Autodesk Inventor part; units mm, degrees
(part 2 of 3)
sketch "Sketch16" plane through (0, 0, -20.23) normal (0, 0, -1) x (-1, 0, 0)
  line L0 (-4.8, 72.125) -> (14.7092, 72.125) construction
  line L1 (-4.8, 51.125) -> (24.7153, 51.125) construction
  line L2 (17.4444, 66.6309) -> (14.7092, 72.125) construction
  line L3 (14.2591, 61.0912) -> (17.4444, 66.6309) construction
  line L4 (20.0758, 56.9365) -> (14.2591, 61.0912) construction
  line L5 (16.752, 54.0974) -> (20.0758, 56.9365) construction
  line L6 (24.7153, 51.125) -> (16.752, 54.0974) construction
  circle A0 centre (-4.8, 5) radius 1.375 construction
  line L7 (-126.5, -2.5) -> (2.5, -2.5) construction
  line L8 (0.5, -0.5) -> (-124.5, -0.5) construction
  line L9 (0.5, -0.5) -> (-124.5, -0.5) construction
  line L10 (-124, 0) -> (0, 0) construction
  line L11 (-124, 0) -> (0, 0) construction
  line L12 (-124, 0) -> (0, 0) construction
  line L13 (0, 0) -> (-122, 0) construction
  line L14 (-122, -0.5) -> (0.5, -0.5) construction
  line L15 (-98.5, 5) -> (-4.8, 5) construction
  line L16 (2.5, 17.7927) -> (-87.0105, 17.7927) construction
  line L17 (2.5, 14.2427) -> (2.5, 16.7927) construction
  line L18 (2.5, 16.7927) -> (2.5, 11.6927) construction
  line L19 (2.5, 10.6927) -> (-87.0105, 10.6927) construction
  line L20 (-37, 78) -> (-37, 22) construction
  line L21 (-40.5, 25.5) -> (-37, 25.5) construction
  line L22 (-40.5, 25.5) -> (-40.5, 74.5) construction
  circle A1 centre (-40.5, 74.5) radius 1.375 construction
  line L23 (-98.5, 25.5) -> (-98.5, 74.5) construction
  line L24 (-42.1, 82.811) -> (-42.1, 78) construction
  line L25 (-122, 78) -> (0, 78) construction
  line L26 (0, 78) -> (-124, 78) construction
  line L27 (2.5, 83.5) -> (-126.5, 83.5) construction
  line L28 (-124.5, 81.5) -> (0.5, 81.5) construction
  line L29 (-124.5, 81.5) -> (0.5, 81.5) construction
  line L30 (0, 81) -> (-124, 81) construction
  line L31 (0, 81) -> (-124, 81) construction
  line L32 (0, 81) -> (-124, 81) construction
  line L33 (-124, 81) -> (0, 81) construction
  line L34 (-124, 81.5) -> (0, 81.5) construction
  line L35 (0, 81) -> (-124, 81) construction
  line L36 (-40.5, 22) -> (-40.5, 25.5) construction
  circle A2 centre (-40.5, 25.5) radius 1.375 construction
  line L37 (-37, 25.5) -> (-37, 22) construction
  line L38 (-37, 22) -> (-40.5, 22) construction
  line L39 (-37, 22) -> (-122, 22) construction
  line L40 (-40.5, 25.5) -> (-98.5, 25.5) construction
  circle A3 centre (-98.5, 74.5) radius 1.375 construction
  line L41 (-122, 78) -> (-124, 78) construction
  line L42 (-122, 22) -> (-122, 78) construction
  line L43 (-98.5, 74.5) -> (-98.5, 5) construction
  line L44 (-124, 81) -> (-124, 0) construction
  line L45 (-124, 81) -> (-124, 0) construction
  line L46 (-122, 0) -> (-122, 78) construction
  line L47 (-124, 78) -> (-124, 0) construction
  line L48 (-124, 78) -> (-124, 81) construction
  line L49 (-124, 81.5) -> (-124.5, 81.5) construction
  line L50 (2.5, 16.7927) -> (2.5, 17.7927) construction
  line L51 (2.5, 11.6927) -> (2.5, 10.6927) construction
  line L52 (-4.8, 6.375) -> (-4.8, 22.1104) construction
  line L53 (-4.8, 5) -> (-4.8, 74.5) construction
  line L54 (0, 78) -> (0, 0) construction
  line L55 (0.5, -0.5) -> (0.5, 78) construction
  line L56 (2.5, -2.5) -> (2.5, 83.5) construction
  line L57 (2.5, 83.5) -> (2.5, -2.5) construction
  line L58 (0.5, 81.5) -> (0.5, -0.5) construction
  line L59 (0.5, 81.5) -> (0.5, -0.5) construction
  line L60 (0, 0) -> (0, 81) construction
  line L61 (0, 0) -> (0, 81) construction
  line L62 (0, 0) -> (0, 81) construction
  circle A4 centre (-98.5, 25.5) radius 1.375 construction
  line L63 (-124, 0) -> (-122, 0) construction
  line L64 (-87.0105, 10.6927) -> (-87.0105, 17.7927) construction
  line L65 (-98.5, 74.5) -> (-168, 74.5) construction
  line L66 (-124, 78) -> (-124, 81) construction
  line L67 (0, 81) -> (0, 78) construction
  line L68 (-4.8, 72.125) -> (-4.8, 51.125) construction
  line L69 (-4.8, 72.125) -> (-4.8, 69.1979) construction
  line L70 (-4.8, 73.125) -> (-4.8, 72.125) construction
  circle A5 centre (-4.8, 74.5) radius 1.375 construction
  line L71 (0, 77.4184) -> (0, 81) construction
  line L72 (0.5, 78) -> (0.5, 81) construction
  line L73 (-81, 78) -> (-81, 90) construction
  line L74 (-53.1, 82.811) -> (-53.1, 78) construction
  line L75 (-47.6, 78) -> (-47.6, 82.811) construction
  line L76 (-47.6, 82.811) -> (-53.1, 82.811) construction
  line L77 (-53.1, 82.811) -> (-42.1, 82.811) construction
  line L78 (-37, 78) -> (-47.6, 78) construction
  line L79 (-37, 78) -> (-69, 78) construction
  line L80 (-57, 90) -> (-57, 78) construction
  line L81 (-55, 92) -> (-55, 83.5) construction
  line L82 (-81, 90) -> (-57, 90) construction
  line L83 (-122, 78) -> (-37, 78) construction
  line L84 (-83, 92) -> (-55, 92) construction
  line L85 (-83, 83.5) -> (-83, 92) construction
  line L86 (-69, 78) -> (-81, 78) construction
  line L87 (0.5, 81.5) -> (-57, 81.5) construction
  line L88 (-53.1, 81.5) -> (-53.1, 83.5) construction
  line L89 (-42.1, 81.5) -> (-42.1, 83.5) construction
  line L90 (-124.5, 81) -> (-126.5, 81) construction
  line L91 (-126.5, -2.5) -> (-126.5, 83.5) construction
  line L92 (0.5, 10.6927) -> (2.5, 10.6927) construction
  line L93 (0.5, 10.6927) -> (0.5, -0.5) construction
  line L94 (0.5, -0.5) -> (-124.5, -0.5) construction
  line L95 (-124.5, -0.5) -> (-124.5, 81.5) construction
  line L96 (-124.5, 81.5) -> (-81, 81.5) construction
  line L97 (-81, 81.5) -> (-81, 90) construction
  line L98 (-81, 90) -> (-57, 90) construction
  line L99 (-57, 90) -> (-57, 81.5) construction
  line L100 (-57, 81.5) -> (0.5, 81.5) construction
  line L101 (0.5, 81.5) -> (0.5, 17.7927) construction
  line L102 (2.5, 17.7927) -> (0.5, 17.7927) construction
  line L103 (2.5, 17.7927) -> (2.5, 83.5) construction
  line L104 (2.5, 83.5) -> (-55, 83.5) construction
  line L105 (-55, 83.5) -> (-55, 92) construction
  line L106 (-55, 92) -> (-83, 92) construction
  line L107 (-83, 92) -> (-83, 83.5) construction
  line L108 (-83, 83.5) -> (-126.5, 83.5) construction
  line L109 (-126.5, 83.5) -> (-126.5, -2.5) construction
  line L110 (-126.5, -2.5) -> (2.5, -2.5) construction
  line L111 (2.5, -2.5) -> (2.5, 10.6927) construction
  line L112 (-122, 22) -> (-124, 22) construction
  line L113 (-124.5, 22) -> (-126.5, 22) construction
  line L114 (-126.5, 83.5) -> (-126.5, 81) construction
  line L115 (-126.5, 22) -> (-126.5, -2.5) construction
  line L116 (-124.5, -0.5) -> (-124.5, 22) construction
  line L117 (-124.5, 81) -> (-124.5, 81.5) construction
  line L118 (-124.5, -0.5) -> (-124.5, 22) construction
  line L119 (-124.5, 81) -> (-124.5, 81.5) construction
  line L120 (0.5, 24.625) -> (0.5, 81.5) projected
  line L121 (2.5, 83.5) -> (2.5, -2.5) projected
  line L122 (0.5, 72.125) -> (2.5, 72.125)
  line L123 (2.5, 72.125) -> (2.5, 51.125)
  line L124 (2.5, 51.125) -> (0.5, 51.125)
  line L125 (0.5, 51.125) -> (0.5, 72.125)
  point P0 (0, 0)
  point P1 (0, 0)
  point P2 (0, 0)
  dimension "d210" = 1
  dimension "d211" = 1
  dimension "d212" = 11
  constraints: 248 end point, 36 point on line, 4 centre point, 4 coincident, 4 parallel, 4 perpendicular, 2 vertical alignment, 1 horizontal, 4 other
  measures "d210" distance of L17.end L16.start
  measures "d211" distance of L18.end L19.start
  measures "d212" distance between parallel lines of L24 L74
extrude "Extrusion14" cut sketch "Sketch16" against normal blind 0.5
sketch "Sketch17" plane through (0, 0, -20.23) normal (0, 0, -1) x (-1, 0, 0)
  line L0 (-53.1, 81.5) -> (-53.1, 83.5) projected
  line L1 (-53.1, 83.5) -> (-55, 83.5) projected
  line L2 (-55, 83.5) -> (-55, 92) projected
  line L3 (-55, 92) -> (-83, 92) projected
  line L4 (-83, 92) -> (-83, 83.5) projected
  line L5 (-83, 83.5) -> (-126.5, 83.5) projected
  line L6 (-126.5, 83.5) -> (-126.5, 76.5) projected
  line L7 (-126.5, 76.5) -> (-124.5, 76.5) projected
  line L8 (-124.5, 76.5) -> (-124.5, 81.5) projected
  line L9 (-124.5, 81.5) -> (-81, 81.5) projected
  line L10 (-81, 81.5) -> (-81, 90) projected
  line L11 (-81, 90) -> (-57, 90) projected
  line L12 (-57, 90) -> (-57, 81.5) projected
  line L13 (-57, 81.5) -> (-53.1, 81.5) projected
  line L14 (2.5, 51.125) -> (0.5, 51.125) projected
  line L15 (0.5, 51.125) -> (0.5, -0.5) projected
  line L16 (0.5, -0.5) -> (-124.5, -0.5) projected
  line L17 (-124.5, -0.5) -> (-124.5, 22) projected
  line L18 (-124.5, 22) -> (-126.5, 22) projected
  line L19 (-126.5, 22) -> (-126.5, -2.5) projected
  line L20 (-126.5, -2.5) -> (2.5, -2.5) projected
  line L21 (2.5, -2.5) -> (2.5, 51.125) projected
  line L22 (0.5, 72.125) -> (2.5, 72.125) projected
  line L23 (2.5, 72.125) -> (2.5, 83.5) projected
  line L24 (2.5, 83.5) -> (-42.1, 83.5) projected
  line L25 (-42.1, 83.5) -> (-42.1, 81.5) projected
  line L26 (-42.1, 81.5) -> (0.5, 81.5) projected
  line L27 (0.5, 81.5) -> (0.5, 72.125) projected
  line L28 (0.5, 72.125) -> (2.5, 72.125) projected
  line L29 (0.5, 51.125) -> (0.5, 72.125) projected
  line L30 (2.5, 51.125) -> (0.5, 51.125) projected
  line L31 (2.5, 72.125) -> (2.5, 51.125) projected
extrude "Extrusion15" add sketch "Sketch17" along normal blind 1.75
sketch "Sketch18" plane through (0, 0, -21.98) normal (0, 0, -1) x (-1, 0, 0)
  line L0 (-53.1, 81.5) -> (-53.1, 83.5) projected
  line L1 (-53.1, 83.5) -> (-55, 83.5) projected
  line L2 (-55, 83.5) -> (-55, 92) projected
  line L3 (-55, 92) -> (-83, 92) projected
  line L4 (-83, 92) -> (-83, 83.5) projected
  line L5 (-83, 83.5) -> (-126.5, 83.5) projected
  line L6 (-124.5, 76.5) -> (-124.5, 81.5) projected
  line L7 (-124.5, 81.5) -> (-81, 81.5) projected
  line L8 (-81, 81.5) -> (-81, 90) construction
  line L9 (-81, 90) -> (-57, 90) construction
  line L10 (-57, 90) -> (-57, 81.5) construction
  line L11 (-57, 81.5) -> (-53.1, 81.5) projected
  line L12 (0.5, 81.5) -> (0.5, -0.5) projected
  line L13 (0.5, -0.5) -> (-124.5, -0.5) projected
  line L14 (-124.5, -0.5) -> (-124.5, 22) projected
  line L15 (-124.5, 22) -> (-126.5, 22) projected
  line L16 (-126.5, 22) -> (-126.5, -2.5) projected
  line L17 (-126.5, -2.5) -> (2.5, -2.5) projected
  line L18 (2.5, -2.5) -> (2.5, 83.5) projected
  line L19 (2.5, 83.5) -> (-42.1, 83.5) projected
  line L20 (-42.1, 83.5) -> (-42.1, 81.5) projected
  line L21 (-42.1, 81.5) -> (0.5, 81.5) projected
  line L22 (-53.1, 81.5) -> (-53.1, 83.5) projected
  line L23 (-42.1, 81.5) -> (-53.1, 81.5) projected
  line L24 (-42.1, 83.5) -> (-42.1, 81.5) projected
  line L25 (-53.1, 83.5) -> (-42.1, 83.5) projected
  line L26 (-124.5, 22) -> (-126.5, 22) projected
  line L27 (-124.5, 76.5) -> (-124.5, 22) projected
  line L28 (-126.5, 22) -> (-126.5, 76.5) projected
  line L29 (-81, 81.5) -> (-57, 81.5)
  line L30 (-126.5, 76.5) -> (-124.5, 76.5) projected
  line L31 (-126.5, 83.5) -> (-126.5, 76.5) projected
  line L32 (-126.5, 76.5) -> (-124.5, 76.5) projected
  point P0 (0, 0)
  constraints: 2 end point, 1 horizontal
extrude "Extrusion16" add sketch "Sketch18" along normal blind 8.5 contours L11 L29 L7 L6 L30 L31 L5 L4 L3 L2 L1 L0 | L0 L25 L20 L23 | L20 L19 L18 L17 L16 L15 L14 L13 L12 L21 | L27 L15 L28 L30
sketch "Sketch20" plane through (0, 0, -30.48) normal (0, 0, -1) x (-1, 0, 0)
  line L0 (-55, 92) -> (-55, 83.5) projected
  line L1 (-83, 92) -> (-55, 92) projected
  line L2 (-55, 83.5) -> (-83, 83.5)
  line L3 (-83, 83.5) -> (-83, 92)
  line L4 (-83, 92) -> (-55, 92)
  line L5 (-55, 92) -> (-55, 83.5)
  point P0 (0, 0)
  constraints: 8 end point, 2 parallel, 1 horizontal, 1 perpendicular
extrude "Extrusion17" cut sketch "Sketch20" against normal blind 6.5
sketch "Sketch21" plane through (0, 0, -30.48) normal (0, 0, -1) x (-1, 0, 0)
  line L0 (-4.8, 72.125) -> (14.7092, 72.125) construction
  line L1 (-4.8, 51.125) -> (24.7153, 51.125) construction
  line L2 (17.4444, 66.6309) -> (14.7092, 72.125) construction
  line L3 (14.2591, 61.0912) -> (17.4444, 66.6309) construction
  line L4 (20.0758, 56.9365) -> (14.2591, 61.0912) construction
  line L5 (16.752, 54.0974) -> (20.0758, 56.9365) construction
  line L6 (24.7153, 51.125) -> (16.752, 54.0974) construction
  circle A0 centre (-4.8, 5) radius 1.375 construction
  line L7 (-126.5, -2.5) -> (2.5, -2.5) construction
  line L8 (-98.5, 5) -> (-4.8, 5) construction
  line L9 (-37, 74.75) -> (-37, 18.75) construction
  line L10 (-40.5, 22.25) -> (-37, 22.25) construction
  line L11 (-40.5, 22.25) -> (-40.5, 71.25) construction
  circle A1 centre (-40.5, 71.25) radius 1.375 construction
  line L12 (-98.5, 22.25) -> (-98.5, 71.25) construction
  line L13 (-42.1, 82.811) -> (-42.1, 74.75) construction
  line L14 (-122, 78) -> (0, 78) construction
  line L15 (0, 78) -> (-124, 78) construction
  line L16 (2.5, 83.5) -> (-126.5, 83.5) construction
  line L17 (-40.5, 18.75) -> (-40.5, 22.25) construction
  circle A2 centre (-40.5, 22.25) radius 1.375 construction
  line L18 (-37, 22.25) -> (-37, 18.75) construction
  line L19 (-37, 18.75) -> (-40.5, 18.75) construction
  line L20 (-37, 22) -> (-122, 22) construction
  line L21 (-40.5, 22.25) -> (-98.5, 22.25) construction
  circle A3 centre (-98.5, 71.25) radius 1.375 construction
  line L22 (-122, 78) -> (-124, 78) construction
  line L23 (-122, 22) -> (-122, 78) construction
  line L24 (-98.5, 74.5) -> (-98.5, 5) construction
  line L25 (-124, 81) -> (-124, 0) construction
  line L26 (-124, 81) -> (-124, 0) construction
  line L27 (-122, 0) -> (-122, 78) construction
  line L28 (-124, 78) -> (-124, 0) construction
  line L29 (-124, 78) -> (-124, 81) construction
  line L30 (-124, 81.5) -> (-124.5, 81.5) construction
  line L31 (2.5, 16.7927) -> (2.5, 17.7927) construction
  line L32 (2.5, 11.6927) -> (2.5, 10.6927) construction
  line L33 (-4.8, 6.375) -> (-4.8, 22.1104) construction
  line L34 (-4.8, 5) -> (-4.8, 74.5) construction
  circle A4 centre (-98.5, 22.25) radius 1.375 construction
  line L35 (-124, 0) -> (-122, 0) construction
  line L36 (-87.0105, 7.4427) -> (-87.0105, 14.5427) construction
  line L37 (-98.5, 74.5) -> (-168, 74.5) construction
  line L38 (-124, 78) -> (-124, 81) construction
  line L39 (-4.8, 72.125) -> (-4.8, 51.125) construction
  line L40 (-4.8, 72.125) -> (-4.8, 69.1979) construction
  line L41 (-4.8, 73.125) -> (-4.8, 72.125) construction
  circle A5 centre (-4.8, 74.5) radius 1.375 construction
  line L42 (-53.1, 82.811) -> (-53.1, 74.75) construction
  line L43 (-47.6, 78) -> (-47.6, 82.811) construction
  line L44 (-47.6, 82.811) -> (-53.1, 82.811) construction
  line L45 (-53.1, 82.811) -> (-42.1, 82.811) construction
  line L46 (-37, 74.75) -> (-47.6, 74.75) construction
  line L47 (-37, 74.75) -> (-69, 74.75) construction
  line L48 (-122, 78) -> (-37, 78) construction
  line L49 (-69, 74.75) -> (-81, 74.75) construction
  line L50 (-53.1, 81.5) -> (-53.1, 83.5)
  line L51 (-42.1, 81.5) -> (-42.1, 83.5)
  line L52 (-124.5, 81) -> (-126.5, 81)
  line L53 (-126.5, -2.5) -> (-126.5, 83.5)
  line L54 (2.5, 17.7927) -> (2.5, 83.5)
  line L55 (2.5, 83.5) -> (-55, 83.5)
  line L56 (-83, 83.5) -> (-126.5, 83.5)
  line L57 (-126.5, 83.5) -> (-126.5, -2.5)
  line L58 (-126.5, -2.5) -> (2.5, -2.5)
  line L59 (2.5, -2.5) -> (2.5, 10.6927)
  line L60 (-126.5, 83.5) -> (-126.5, 81) construction
  line L61 (-126.5, 22) -> (-126.5, -2.5) construction
  line L62 (-124.5, -0.5) -> (-124.5, 22) construction
  line L63 (-124.5, 81) -> (-124.5, 81.5) construction
  line L64 (-124.5, -0.5) -> (-124.5, 22) construction
  line L65 (-124.5, 81) -> (-124.5, 81.5) construction
  line L66 (-124, 81) -> (-3.3, 81) construction
  line L67 (-3.3, 81) -> (-8.3, 81) construction
  line L68 (-8.3, 81) -> (-119, 81) construction
  line L69 (-8.3, 81) -> (-8.3, -29.8281) construction
  line L70 (-119, 81) -> (-119, -36.294) construction
  line L71 (-119, 81) -> (-119, 78.9) construction
  line L72 (-119, 75.65) -> (-8.3, 75.65) construction
  line L73 (-119, 75.65) -> (-119, 8.25) construction
  line L74 (-119, 8.25) -> (-8.3, 8.25) construction
  line L75 (-119, 75.65) -> (-8.3, 75.65) construction
  line L76 (-8.3, 8.25) -> (-119, 8.25) construction
  line L77 (-119, 8.25) -> (-119, 75.65) construction
  line L78 (-83, 83.5) -> (-83, 92) projected
  line L79 (-83, 83.5) -> (-55, 83.5)
  line L80 (2.5, 17.7927) -> (2.5, 10.6927)
  line L81 (2.5, -2.5) -> (2.5, 83.5) projected
  line L82 (29.5237, 30.2885) -> (29.5237, 27.0385)
  line L83 (-8.3, 75.65) -> (-4.3, 75.65)
  line L84 (-8.3, 75.65) -> (-4.3, 75.65) construction
  line L85 (-8.3, 8.25) -> (-4.3, 8.25) construction
  line L86 (-8.3, 8.25) -> (-4.3, 8.25) construction
  line L87 (-4.3, 8.25) -> (-4.3, 75.65) construction
  line L88 (-119, 75.65) -> (-4.3, 75.65)
  line L89 (-4.3, 75.65) -> (-4.3, 8.25)
  line L90 (-4.3, 8.25) -> (-119, 8.25)
  line L91 (-119, 8.25) -> (-119, 75.65)
  dimension "d226" = 11
  dimension "d227" = 120.7
  dimension "d228" = 5
  dimension "d229" = 110.7
  dimension "d231" = 2.1
  dimension "d232" = 67.4
  dimension "d1063" = 3.25
  dimension "d1064" = 4
  dimension "d1065" = 0
  dimension "d1067" = 0
  constraints: 180 end point, 16 point on line, 6 horizontal, 4 centre point, 4 coincident, 4 parallel, 4 perpendicular, 3 collinear, 2 vertical, 2 vertical alignment, 4 other
  measures "d226" distance between parallel lines of L13 L42
  measures "d227" distance of L66.start L66.end
  measures "d228" distance of L66.end L67.end
  measures "d229" distance of L67.end L68.end
  measures "d231" distance of L71.end L68.end
  measures "d232" distance of L72.start L73.end
  measures "d1063" distance of L82.start L82.end
  measures "d1064" distance of L75.end L83.end
  measures "d1065" distance between parallel lines of L83 L84
  measures "d1067" distance between parallel lines of L85 L86
extrude "Extrusion18" add sketch "Sketch21" along normal blind 2
sketch "Sketch29" plane through (0, 0, 0) normal (0, 0, -1) x (-1, 0, 0)
  line L0 (-94.5, 81.5) -> (-114.5, 81.5)
  line L1 (-114.5, 83.5) -> (-114.5, 81.5)
  line L2 (-124.5, 83.5) -> (-114.5, 83.5)
  line L3 (-124.5, 83.5) -> (-124.5, 81.5)
  line L4 (-124.5, 81.5) -> (-124.5, -0.5)
  line L5 (-124.5, -2.5) -> (-124.5, -0.5)
  line L6 (-114.5, -2.5) -> (-124.5, -2.5)
  line L7 (-114.5, -2.5) -> (-114.5, -0.5)
  line L8 (-114.5, -0.5) -> (-94.5, -0.5)
  line L9 (-94.5, -2.5) -> (-94.5, -0.5)
  line L10 (-84.5, -2.5) -> (-94.5, -2.5)
  line L11 (-84.5, -2.5) -> (-84.5, -0.5)
  line L12 (-84.5, -0.5) -> (-64.5, -0.5)
  line L13 (-64.5, -2.5) -> (-64.5, -0.5)
  line L14 (-54.5, -2.5) -> (-64.5, -2.5)
  line L15 (-54.5, -2.5) -> (-54.5, -0.5)
  line L16 (-54.5, -0.5) -> (-34.5, -0.5)
  line L17 (-34.5, -2.5) -> (-34.5, -0.5)
  line L18 (-24.5, -2.5) -> (-34.5, -2.5)
  line L19 (-24.5, -2.5) -> (-24.5, -0.5)
  line L20 (-24.5, -0.5) -> (-4.5, -0.5)
  line L21 (-4.5, -2.5) -> (-4.5, -0.5)
  line L22 (0.5, -2.5) -> (-4.5, -2.5)
  line L23 (0.5, -2.5) -> (0.5, 10.6927)
  line L24 (0.5, 10.6927) -> (-87.0105, 10.6927)
  line L25 (-87.0105, 10.6927) -> (-87.0105, 17.7927)
  line L26 (-87.0105, 17.7927) -> (-4.5, 17.7927)
  line L27 (-4.5, 17.7927) -> (-4.5, 24.0927)
  line L28 (-4.5, 24.0927) -> (-2.5, 24.0927)
  line L29 (-2.5, 24.0927) -> (-2.5, 24.125)
  line L30 (-2.5, 24.125) -> (0.5, 24.125)
  line L31 (0.5, 24.125) -> (0.5, 83.5)
  line L32 (-4.5, 83.5) -> (0.5, 83.5)
  line L33 (-4.5, 83.5) -> (-4.5, 81.5)
  line L34 (-4.5, 81.5) -> (-24.5, 81.5)
  line L35 (-24.5, 83.5) -> (-24.5, 81.5)
  line L36 (-34.5, 83.5) -> (-24.5, 83.5)
  line L37 (-34.5, 83.5) -> (-34.5, 81.5)
  line L38 (-34.5, 81.5) -> (-57, 81.5)
  line L39 (-57, 81.5) -> (-57, 90)
  line L40 (-57, 90) -> (-81, 90)
  line L41 (-81, 90) -> (-81, 81.5)
  line L42 (-81, 81.5) -> (-84.5, 81.5)
  line L43 (-84.5, 83.5) -> (-84.5, 81.5)
  line L44 (-94.5, 83.5) -> (-84.5, 83.5)
  line L45 (-94.5, 83.5) -> (-94.5, 81.5)
  circle A0 centre (-98.5, 5) radius 3.8038
  circle A1 centre (-4.8, 74.5) radius 3.8038
  circle A2 centre (-98.5, 74.5) radius 3.8038
  circle A3 centre (-40.5, 74.5) radius 3.8038
  circle A4 centre (-40.5, 25.5) radius 3.8038
  circle A5 centre (-98.5, 25.5) radius 3.8038
  circle A6 centre (-4.8, 5) radius 3.8038
  line L46 (-80.4572, 45.3554) -> (-80.4572, 50.3554)
  line L47 (-80.4572, 50.3554) -> (-80.4572, 60.3554)
  line L48 (-80.4572, 50.3554) -> (-76.127, 47.8554)
  line L49 (-76.127, 47.8554) -> (-76.127, 42.8554)
  line L50 (-76.127, 42.8554) -> (-80.4572, 40.3554)
  line L51 (-80.4572, 40.3554) -> (-84.7873, 42.8554)
  line L52 (-84.7873, 42.8554) -> (-84.7873, 47.8554)
  line L53 (-84.7873, 47.8554) -> (-80.4572, 50.3554)
  line L54 (-80.4572, 70.3554) -> (-80.4572, 80.3554)
  line L55 (-80.4572, 70.3554) -> (-76.127, 67.8554)
  line L56 (-84.7873, 67.8554) -> (-80.4572, 70.3554)
  line L57 (-80.4572, 65.3554) -> (-80.4572, 70.3554)
  line L58 (-76.127, 67.8554) -> (-76.127, 62.8554)
  line L59 (-84.7873, 62.8554) -> (-84.7873, 67.8554)
  line L60 (-80.4572, 60.3554) -> (-84.7873, 62.8554)
  line L61 (-76.127, 62.8554) -> (-80.4572, 60.3554)
  line L62 (-76.127, 47.8554) -> (-66.127, 47.8554)
  line L63 (-66.127, 47.8554) -> (-66.127, 55.3554)
  line L64 (-84.7873, 45.3554) -> (-92.0042, 45.3554)
  line L65 (-61.7969, 70.3554) -> (-66.127, 72.8554)
  line L66 (-57.4668, 77.8554) -> (-57.4668, 72.8554)
  line L67 (-66.127, 72.8554) -> (-66.127, 77.8554)
  line L68 (-61.7969, 80.3554) -> (-57.4668, 77.8554)
  line L69 (-66.127, 77.8554) -> (-61.7969, 80.3554)
  line L70 (-61.7969, 75.3554) -> (-61.7969, 80.3554)
  line L71 (-57.4668, 72.8554) -> (-61.7969, 70.3554)
  line L72 (-61.7969, 55.3554) -> (-61.7969, 60.3554)
  line L73 (-61.7969, 60.3554) -> (-61.7969, 70.3554)
  line L74 (-47.4668, 57.8554) -> (-47.4668, 65.3554)
  line L75 (-57.4668, 57.8554) -> (-47.4668, 57.8554)
  line L76 (-61.7969, 60.3554) -> (-57.4668, 57.8554)
  line L77 (-66.127, 57.8554) -> (-61.7969, 60.3554)
  line L78 (-66.127, 55.3554) -> (-73.3439, 55.3554)
  line L79 (-57.4668, 57.8554) -> (-57.4668, 52.8554)
  line L80 (-66.127, 52.8554) -> (-66.127, 57.8554)
  line L81 (-61.7969, 50.3554) -> (-66.127, 52.8554)
  line L82 (-57.4668, 52.8554) -> (-61.7969, 50.3554)
  line L83 (-43.1366, 65.3554) -> (-43.1366, 70.3554)
  line L84 (-43.1366, 70.3554) -> (-43.1366, 80.3554)
  line L85 (-28.8065, 67.8554) -> (-28.8065, 75.3554)
  line L86 (-38.8065, 67.8554) -> (-28.8065, 67.8554)
  line L87 (-43.1366, 70.3554) -> (-38.8065, 67.8554)
  line L88 (-47.4668, 67.8554) -> (-43.1366, 70.3554)
  line L89 (-47.4668, 65.3554) -> (-54.6837, 65.3554)
  line L90 (-38.8065, 67.8554) -> (-38.8065, 62.8554)
  line L91 (-47.4668, 62.8554) -> (-47.4668, 67.8554)
  line L92 (-43.1366, 60.3554) -> (-47.4668, 62.8554)
  line L93 (-38.8065, 62.8554) -> (-43.1366, 60.3554)
  line L94 (-24.4764, 75.3554) -> (-24.4764, 80.3554)
  line L95 (-20.1463, 77.8554) -> (-10.1463, 77.8554)
  line L96 (-24.4764, 80.3554) -> (-20.1463, 77.8554)
  line L97 (-28.8065, 77.8554) -> (-24.4764, 80.3554)
  line L98 (-20.1463, 77.8554) -> (-20.1463, 72.8554)
  line L99 (-20.1463, 72.8554) -> (-24.4764, 70.3554)
  line L100 (-24.4764, 70.3554) -> (-28.8065, 72.8554)
  line L101 (-28.8065, 72.8554) -> (-28.8065, 77.8554)
  line L102 (-28.8065, 75.3554) -> (-36.0234, 75.3554)
  line L103 (-80.4572, 10.3554) -> (-80.4572, 20.3554)
  line L104 (-76.127, 27.8554) -> (-76.127, 22.8554)
  line L105 (-76.127, 22.8554) -> (-80.4572, 20.3554)
  line L106 (-80.4572, 20.3554) -> (-84.7873, 22.8554)
  line L107 (-80.4572, 30.3554) -> (-76.127, 27.8554)
  line L108 (-80.4572, 25.3554) -> (-80.4572, 30.3554)
  line L109 (-84.7873, 22.8554) -> (-84.7873, 27.8554)
  line L110 (-84.7873, 27.8554) -> (-80.4572, 30.3554)
  line L111 (-80.4572, 0.3554) -> (-84.7873, 2.8554)
  line L112 (-84.7873, 2.8554) -> (-84.7873, 7.8554)
  line L113 (-76.127, 7.8554) -> (-76.127, 2.8554)
  line L114 (-84.7873, 7.8554) -> (-80.4572, 10.3554)
  line L115 (-80.4572, 5.3554) -> (-80.4572, 10.3554)
  line L116 (-80.4572, 10.3554) -> (-76.127, 7.8554)
  line L117 (-76.127, 2.8554) -> (-80.4572, 0.3554)
  line L118 (-61.7969, 40.3554) -> (-61.7969, 50.3554)
  line L119 (-66.127, 37.8554) -> (-61.7969, 40.3554)
  line L120 (-61.7969, 40.3554) -> (-57.4668, 37.8554)
  line L121 (-61.7969, 35.3554) -> (-61.7969, 40.3554)
  line L122 (-80.4572, 30.3554) -> (-80.4572, 40.3554)
  line L123 (-66.127, 32.8554) -> (-66.127, 37.8554)
  line L124 (-61.7969, 30.3554) -> (-66.127, 32.8554)
  line L125 (-57.4668, 32.8554) -> (-61.7969, 30.3554)
  line L126 (-57.4668, 37.8554) -> (-57.4668, 32.8554)
  line L127 (-61.7969, 20.3554) -> (-61.7969, 30.3554)
  line L128 (-66.127, 12.8554) -> (-66.127, 17.8554)
  line L129 (-66.127, 17.8554) -> (-61.7969, 20.3554)
  line L130 (-61.7969, 15.3554) -> (-61.7969, 20.3554)
  line L131 (-61.7969, 20.3554) -> (-57.4668, 17.8554)
  line L132 (-61.7969, 10.3554) -> (-66.127, 12.8554)
  line L133 (-57.4668, 17.8554) -> (-57.4668, 12.8554)
  line L134 (-57.4668, 12.8554) -> (-61.7969, 10.3554)
  line L135 (-66.127, -4.6446) -> (-73.3439, -4.6446)
  line L136 (-66.127, -2.1446) -> (-61.7969, 0.3554)
  line L137 (-61.7969, -4.6446) -> (-61.7969, 0.3554)
  line L138 (-61.7969, 0.3554) -> (-57.4668, -2.1446)
  line L139 (-43.1366, 50.3554) -> (-43.1366, 60.3554)
  line L140 (-24.4764, 40.3554) -> (-24.4764, 50.3554)
  line L141 (-38.8065, 47.8554) -> (-38.8065, 42.8554)
  line L142 (-43.1366, 45.3554) -> (-43.1366, 50.3554)
  line L143 (-47.4668, 47.8554) -> (-43.1366, 50.3554)
  line L144 (-38.8065, 42.8554) -> (-43.1366, 40.3554)
  line L145 (-47.4668, 42.8554) -> (-47.4668, 47.8554)
  line L146 (-43.1366, 40.3554) -> (-47.4668, 42.8554)
  line L147 (-43.1366, 50.3554) -> (-38.8065, 47.8554)
  line L148 (-43.1366, 20.3554) -> (-47.4668, 22.8554)
  line L149 (-38.8065, 27.8554) -> (-38.8065, 22.8554)
  line L150 (-43.1366, 10.3554) -> (-43.1366, 20.3554)
  line L151 (-38.8065, 7.8554) -> (-28.8065, 7.8554)
  line L152 (-28.8065, 7.8554) -> (-28.8065, 15.3554)
  line L153 (-28.8065, 15.3554) -> (-36.0234, 15.3554)
  line L154 (-28.8065, 12.8554) -> (-28.8065, 17.8554)
  line L155 (-38.8065, 22.8554) -> (-43.1366, 20.3554)
  line L156 (-47.4668, 27.8554) -> (-43.1366, 30.3554)
  line L157 (-43.1366, 25.3554) -> (-43.1366, 30.3554)
  line L158 (-43.1366, 30.3554) -> (-38.8065, 27.8554)
  line L159 (-47.4668, 22.8554) -> (-47.4668, 27.8554)
  line L160 (-1.486, 67.8554) -> (-1.486, 62.8554)
  line L161 (-1.486, 62.8554) -> (-5.8161, 60.3554)
  line L162 (-5.8161, 70.3554) -> (-1.486, 67.8554)
  line L163 (-5.8161, 65.3554) -> (-5.8161, 70.3554)
  line L164 (-10.1463, 67.8554) -> (-5.8161, 70.3554)
  line L165 (-10.1463, 62.8554) -> (-10.1463, 67.8554)
  line L166 (-5.8161, 60.3554) -> (-10.1463, 62.8554)
  line L167 (-5.8161, 50.3554) -> (-5.8161, 60.3554)
  line L168 (-5.8161, 50.3554) -> (-1.486, 47.8554)
  line L169 (-24.4764, 15.3554) -> (-24.4764, 20.3554)
  line L170 (-24.4764, 20.3554) -> (-24.4764, 30.3554)
  line L171 (-10.1463, 25.3554) -> (-17.3631, 25.3554)
  line L172 (-28.8065, 17.8554) -> (-24.4764, 20.3554)
  line L173 (-24.4764, 20.3554) -> (-20.1463, 17.8554)
  line L174 (-10.1463, 17.8554) -> (-10.1463, 25.3554)
  line L175 (-20.1463, 17.8554) -> (-20.1463, 12.8554)
  line L176 (-24.4764, 10.3554) -> (-28.8065, 12.8554)
  line L177 (-20.1463, 12.8554) -> (-24.4764, 10.3554)
  line L178 (-20.1463, 17.8554) -> (-10.1463, 17.8554)
  line L179 (-61.7969, 0.3554) -> (-61.7969, 10.3554)
  line L180 (-47.4668, 5.3554) -> (-54.6837, 5.3554)
  line L181 (-57.4668, -2.1446) -> (-47.4668, -2.1446)
  line L182 (-47.4668, 7.8554) -> (-43.1366, 10.3554)
  line L183 (-43.1366, 5.3554) -> (-43.1366, 10.3554)
  line L184 (-47.4668, -2.1446) -> (-47.4668, 5.3554)
  line L185 (-43.1366, 10.3554) -> (-38.8065, 7.8554)
  line L186 (-43.1366, 0.3554) -> (-47.4668, 2.8554)
  line L187 (-38.8065, 7.8554) -> (-38.8065, 2.8554)
  line L188 (-38.8065, 2.8554) -> (-43.1366, 0.3554)
  line L189 (-47.4668, 2.8554) -> (-47.4668, 7.8554)
  line L190 (-43.1366, 30.3554) -> (-43.1366, 40.3554)
  line L191 (-20.1463, 32.8554) -> (-24.4764, 30.3554)
  line L192 (-24.4764, 30.3554) -> (-28.8065, 32.8554)
  line L193 (-20.1463, 37.8554) -> (-20.1463, 32.8554)
  line L194 (-24.4764, 40.3554) -> (-20.1463, 37.8554)
  line L195 (-28.8065, 32.8554) -> (-28.8065, 37.8554)
  line L196 (-24.4764, 35.3554) -> (-24.4764, 40.3554)
  line L197 (-28.8065, 37.8554) -> (-24.4764, 40.3554)
  line L198 (-10.1463, 22.8554) -> (-10.1463, 27.8554)
  line L199 (-10.1463, 27.8554) -> (-5.8161, 30.3554)
  line L200 (-5.8161, 20.3554) -> (-10.1463, 22.8554)
  line L201 (-5.8161, 30.3554) -> (-5.8161, 40.3554)
  line L202 (-5.8161, 30.3554) -> (-1.486, 27.8554)
  line L203 (-5.8161, 25.3554) -> (-5.8161, 30.3554)
  line L204 (-1.486, 22.8554) -> (-5.8161, 20.3554)
  line L205 (-1.486, 27.8554) -> (-1.486, 22.8554)
  line L206 (-1.486, 42.8554) -> (-5.8161, 40.3554)
  line L207 (-5.8161, 40.3554) -> (-10.1463, 42.8554)
  line L208 (-1.486, 47.8554) -> (-1.486, 42.8554)
  line L209 (-10.1463, 42.8554) -> (-10.1463, 47.8554)
  line L210 (-5.8161, 45.3554) -> (-5.8161, 50.3554)
  line L211 (-10.1463, 47.8554) -> (-5.8161, 50.3554)
  line L212 (-28.8065, 52.8554) -> (-28.8065, 57.8554)
  line L213 (-20.1463, 52.8554) -> (-24.4764, 50.3554)
  line L214 (-24.4764, 55.3554) -> (-24.4764, 60.3554)
  line L215 (-28.8065, 57.8554) -> (-24.4764, 60.3554)
  line L216 (-20.1463, 57.8554) -> (-20.1463, 52.8554)
  line L217 (-24.4764, 60.3554) -> (-24.4764, 70.3554)
  line L218 (-24.4764, 60.3554) -> (-20.1463, 57.8554)
  line L219 (-24.4764, 50.3554) -> (-28.8065, 52.8554)
  line L220 (-5.8161, 70.3554) -> (-5.8161, 80.3554)
  line L221 (-99.1174, 77.8554) -> (-103.4475, 80.3554)
  line L222 (-94.7873, 80.3554) -> (-99.1174, 77.8554)
  line L223 (-122.1078, 32.8554) -> (-129.3247, 32.8554)
  line L224 (-132.1078, 25.3554) -> (-122.1078, 25.3554)
  line L225 (-117.7777, 32.8554) -> (-117.7777, 37.8554)
  line L226 (-113.4475, 30.3554) -> (-117.7777, 27.8554)
  line L227 (-122.1078, 35.3554) -> (-117.7777, 37.8554)
  line L228 (-122.1078, 30.3554) -> (-122.1078, 35.3554)
  line L229 (-117.7777, 27.8554) -> (-122.1078, 30.3554)
  line L230 (-122.1078, 25.3554) -> (-122.1078, 32.8554)
  line L231 (-113.4475, 35.3554) -> (-113.4475, 30.3554)
  line L232 (-117.7777, 37.8554) -> (-113.4475, 35.3554)
  line L233 (-117.7777, 37.8554) -> (-117.7777, 47.8554)
  line L234 (-113.4475, 35.3554) -> (-103.4475, 35.3554)
  line L235 (-103.4475, 42.8554) -> (-110.6644, 42.8554)
  line L236 (-103.4475, 35.3554) -> (-103.4475, 42.8554)
  line L237 (-99.1174, 37.8554) -> (-103.4475, 40.3554)
  line L238 (-103.4475, 40.3554) -> (-103.4475, 45.3554)
  line L239 (-103.4475, 45.3554) -> (-99.1174, 47.8554)
  line L240 (-99.1174, 42.8554) -> (-99.1174, 47.8554)
  line L241 (-94.7873, 45.3554) -> (-94.7873, 40.3554)
  line L242 (-99.1174, 47.8554) -> (-94.7873, 45.3554)
  line L243 (-84.7873, 45.3554) -> (-84.7873, 52.8554)
  line L244 (-94.7873, 45.3554) -> (-84.7873, 45.3554)
  line L245 (-99.1174, 27.8554) -> (-99.1174, 37.8554)
  line L246 (-94.7873, 40.3554) -> (-99.1174, 37.8554)
  line L247 (-99.1174, 47.8554) -> (-99.1174, 57.8554)
  line L248 (-113.4475, 50.3554) -> (-117.7777, 47.8554)
  line L249 (-117.7777, 47.8554) -> (-122.1078, 50.3554)
  line L250 (-113.4475, 55.3554) -> (-113.4475, 50.3554)
  line L251 (-122.1078, 50.3554) -> (-122.1078, 55.3554)
  line L252 (-117.7777, 52.8554) -> (-117.7777, 57.8554)
  line L253 (-117.7777, 57.8554) -> (-113.4475, 55.3554)
  line L254 (-122.1078, 55.3554) -> (-117.7777, 57.8554)
  line L255 (-103.4475, 65.3554) -> (-99.1174, 67.8554)
  line L256 (-99.1174, 67.8554) -> (-94.7873, 65.3554)
  line L257 (-99.1174, 62.8554) -> (-99.1174, 67.8554)
  line L258 (-94.7873, 65.3554) -> (-94.7873, 60.3554)
  line L259 (-94.7873, 60.3554) -> (-99.1174, 57.8554)
  line L260 (-103.4475, 60.3554) -> (-103.4475, 65.3554)
  line L261 (-99.1174, 57.8554) -> (-103.4475, 60.3554)
  line L262 (-117.7777, 57.8554) -> (-117.7777, 67.8554)
  line L263 (-99.1174, 67.8554) -> (-99.1174, 77.8554)
  line L264 (-117.7777, 77.8554) -> (-113.4475, 75.3554)
  line L265 (-117.7777, 72.8554) -> (-117.7777, 77.8554)
  line L266 (-122.1078, 75.3554) -> (-117.7777, 77.8554)
  line L267 (-113.4475, 70.3554) -> (-117.7777, 67.8554)
  line L268 (-122.1078, 70.3554) -> (-122.1078, 75.3554)
  line L269 (-117.7777, 67.8554) -> (-122.1078, 70.3554)
  line L270 (-113.4475, 75.3554) -> (-113.4475, 70.3554)
  line L271 (-122.1078, -4.6446) -> (-117.7777, -2.1446)
  line L272 (-117.7777, -2.1446) -> (-113.4475, -4.6446)
  line L273 (-103.4475, 25.3554) -> (-99.1174, 27.8554)
  line L274 (-99.1174, 22.8554) -> (-99.1174, 27.8554)
  line L275 (-117.7777, 17.8554) -> (-117.7777, 27.8554)
  line L276 (-103.4475, 20.3554) -> (-103.4475, 25.3554)
  line L277 (-94.7873, 25.3554) -> (-94.7873, 20.3554)
  line L278 (-99.1174, 17.8554) -> (-103.4475, 20.3554)
  line L279 (-94.7873, 20.3554) -> (-99.1174, 17.8554)
  line L280 (-99.1174, 27.8554) -> (-94.7873, 25.3554)
  line L281 (-99.1174, 7.8554) -> (-99.1174, 17.8554)
  line L282 (-99.1174, -2.1446) -> (-103.4475, 0.3554)
  line L283 (-94.7873, 0.3554) -> (-99.1174, -2.1446)
  line L284 (-94.7873, 5.3554) -> (-94.7873, 0.3554)
  line L285 (-99.1174, 7.8554) -> (-94.7873, 5.3554)
  line L286 (-99.1174, 2.8554) -> (-99.1174, 7.8554)
  line L287 (-103.4475, 0.3554) -> (-103.4475, 5.3554)
  line L288 (-103.4475, 5.3554) -> (-99.1174, 7.8554)
  line L289 (-117.7777, -2.1446) -> (-117.7777, 7.8554)
  line L290 (-113.4475, 10.3554) -> (-117.7777, 7.8554)
  line L291 (-117.7777, 7.8554) -> (-122.1078, 10.3554)
  line L292 (-113.4475, 15.3554) -> (-113.4475, 10.3554)
  line L293 (-122.1078, 10.3554) -> (-122.1078, 15.3554)
  line L294 (-117.7777, 17.8554) -> (-113.4475, 15.3554)
  line L295 (-117.7777, 12.8554) -> (-117.7777, 17.8554)
  line L296 (-122.1078, 15.3554) -> (-117.7777, 17.8554)
  point P0 (0, 0)
  point P1 (-124.5, 4.2179)
  point P2 (-124.5, 49.2179)
  dimension "d995" = 5
  dimension "d996" = 10
  dimension "d997" = 5
  dimension "d998" = 10
  dimension "d999" = 5
  dimension "d1000" = 10
  dimension "d1001" = 5
  dimension "d1002" = 5
  dimension "d1003" = 10
  dimension "d1004" = 5
  dimension "d1005" = 5
  dimension "d1006" = 10
  dimension "d1007" = 5
  dimension "d1008" = 10
  dimension "d1009" = 5
  dimension "d1010" = 10
  dimension "d1011" = 5
  dimension "d1012" = 10
  dimension "d1013" = 5
  dimension "d1014" = 10
  dimension "d1015" = 5
  dimension "d1016" = 10
  dimension "d1017" = 5
  dimension "d1018" = 10
  dimension "d1019" = 5
  dimension "d1020" = 10
  dimension "d1021" = 5
  dimension "d1022" = 10
  dimension "d1023" = 5
  dimension "d1024" = 10
  dimension "d1025" = 5
  dimension "d1026" = 10
  dimension "d1027" = 5
  dimension "d1028" = 5
  dimension "d1029" = 5
  dimension "d1030" = 5
  dimension "d1031" = 10
  dimension "d1032" = 5
  dimension "d1033" = 10
  dimension "d1034" = 5
  dimension "d1035" = 5
  dimension "d1036" = 10
  dimension "d1037" = 5
  dimension "d1038" = 10
  dimension "d1039" = 10
  dimension "d1040" = 5
  dimension "d1041" = 10
  dimension "d1042" = 5
  dimension "d1043" = 10
  dimension "d1044" = 5
  dimension "d1045" = 10
  constraints: 594 end point, 28 coincident, 28 vertical, 27 point on line, 20 horizontal, 9 midpoint, 7 centre point, 355 other
  measures "d995" distance of L46.start L46.end
  measures "d996" distance of L46.end L47.end
  measures "d997" distance of L57.start L55.start
  measures "d998" distance of L55.start L54.end
  measures "d999" distance of L72.start L73.start
  measures "d1000" distance of L73.start L73.end
  measures "d1001" distance of L70.start L68.start
  measures "d1002" distance of L83.start L88.end
  measures "d1003" distance of L88.end L84.end
  measures "d1004" distance of L94.start L96.start
  measures "d1005" distance of L115.start L114.end
  measures "d1006" distance of L114.end L103.end
  measures "d1007" distance of L108.start L122.start
  measures "d1008" distance of L122.start L122.end
  measures "d1009" distance of L137.start L137.end
  measures "d1010" distance of L137.end L179.end
  measures "d1011" distance of L130.start L127.start
  measures "d1012" distance of L127.start L127.end
  measures "d1013" distance of L121.start L118.start
  measures "d1014" distance of L118.start L118.end
  measures "d1015" distance of L183.start L182.end
  measures "d1016" distance of L182.end L150.end
  measures "d1017" distance of L157.start L190.start
  measures "d1018" distance of L190.start L190.end
  measures "d1019" distance of L142.start L142.end
  measures "d1020" distance of L142.end L139.end
  measures "d1021" distance of L169.start L169.end
  measures "d1022" distance of L169.end L170.end
  measures "d1023" distance of L196.start L140.start
  measures "d1024" distance of L140.start L140.end
  measures "d1025" distance of L214.start L217.start
  measures "d1026" distance of L217.start L217.end
  measures "d1027" distance of L203.start L201.start
  measures "d1028" distance of L210.start L167.start
  measures "d1029" distance of L163.start L164.end
  measures "d1030" distance of L225.start L233.start
  measures "d1031" distance of L233.start L233.end
  measures "d1032" distance of L252.start L253.start
  measures "d1033" distance of L253.start L262.end
  measures "d1034" distance of L265.start L265.end
  measures "d1035" distance of L240.start L242.start
  measures "d1036" distance of L242.start L247.end
  measures "d1037" distance of L257.start L263.start
  measures "d1038" distance of L263.start L263.end
  measures "d1039" distance of L271.end L289.end
  measures "d1040" distance of L295.start L294.start
  measures "d1041" distance of L294.start L275.end
  measures "d1042" distance of L286.start L281.start
  measures "d1043" distance of L281.start L281.end
  measures "d1044" distance of L274.start L273.end
  measures "d1045" distance of L273.end L245.end
extrude "Extrusion25" cut sketch "Sketch29" against normal blind 3 contours L228 L227 L232 L231 L226 L229 | L294 L292 L290 L291 L293 L296 | L236 L238 L239 L242 L241 L246 L237 | L52 L53 L48 L49 L50 L51 | L107 L104 L105 L106 L109 L110 | L63 L80 L77 L76 L79 L82 L81 | L120 L126 L125 L124 L123 L119 | L192 L195 L197 L194 L193 L191 | L185 L187 L188 L186 L184 L189 L182 | L74 L91 L88 L87 L90 L93 L92 | L219 L212 L215 L218 L216 L213 | L147 L141 L144 L146 L145 L143 | L85 L101 L97 L96 L98 L99 L100 | L55 L58 L61 L60 L59 L56 | L65 L67 L69 L68 L66 L71 | L111 L112 L114 L116 L113 L117 | L160 L161 L166 L165 L164 L162 | L168 L208 L206 L207 L209 L211 | L248 L249 L251 L254 L253 L250 | L255 L256 L258 L259 L261 L260 | L264 L270 L267 L269 L268 L266
sketch "Sketch33" plane through (87.0105, 10.6927, 0) normal (1, 0, 0) x (0, 0, -1)
  line L0 (0, 0) -> (0, 7.1) projected
  line L1 (0, 0) -> (6, 0) projected
  line L2 (6, 7.1) -> (6, 0) projected
  line L3 (0, 7.1) -> (6, 7.1) projected
  line L4 (6, 7.1) -> (6, 0) projected
  line L5 (6, 7.1) -> (6.5, 7.1) construction
  line L6 (6.5, 7.1) -> (6.5, 7.6) construction
  line L7 (6.5, 7.6) -> (6, 7.6) construction
  line L8 (6, 7.6) -> (6, 7.1) construction
  line L9 (0, 0) -> (6, 0) construction
  line L10 (6, 0) -> (6.5, 0) construction
  line L11 (6.5, 0) -> (6.5, -0.5) construction
  line L12 (6.5, -0.5) -> (6, -0.5) construction
  line L13 (6, -0.5) -> (6, 0) construction
  line L14 (0, 13.9323) -> (0, 0) projected
  line L15 (6.5, 7.6) -> (0, 7.6)
  line L16 (0, 7.6) -> (0, -0.5)
  line L17 (0, -0.5) -> (6.5, -0.5)
  line L18 (6.5, -0.5) -> (6.5, 7.6)
  line L19 (0, 7.1) -> (6, 7.1)
  line L20 (6, 7.1) -> (6, 0)
  line L21 (6, 0) -> (0, 0)
  line L22 (0, 0) -> (0, 7.1)
  point P0 (0, -10.6927)
  point P1 (0, -13.1927)
  dimension "d1054" = 0.5
  dimension "d1055" = 0.5
  dimension "d1056" = 0.5
  dimension "d1057" = 0.5
  constraints: 32 end point, 8 parallel, 4 perpendicular, 3 horizontal, 1 point on line
  measures "d1054" distance of L7.end L6.end
  measures "d1055" distance of L6.end L5.end
  measures "d1056" distance of L11.end L12.end
  measures "d1057" distance of L10.end L11.end
extrude "Extrusion27" add sketch "Sketch33" against normal blind 87.511 contours L1 L2 L3 L14 L15 L18 L17 L16
sketch "Sketch34" plane through (-0.5005, 10.6927, 0) normal (-1, 0, 0) x (0, 0, 1)
  line L0 (-6.5, 6.3) -> (-6, 6.3) projected
  line L1 (-6.5, 6.3) -> (-6.5, 0.8) projected
  line L2 (-6, 0.8) -> (-6.5, 0.8) projected
  line L3 (-6, 0.8) -> (-6, 6.3) projected
  point P0 (0, -10.6927)
extrude "Extrusion28" cut sketch "Sketch34" against normal blind 12
sketch "Sketch35" plane through (98.5, 74.5, -3) normal (0, 0, -1) x (-1, 0, 0)
  circle A0 centre (92.45, 0) radius 1.375 projected
  circle A1 centre (92.45, 0) radius 3 projected
  circle A2 centre (92.45, -69.5) radius 1.375 projected
  circle A3 centre (92.45, -69.5) radius 3 projected
  circle A4 centre (0, -69.5) radius 1.375 projected
  circle A5 centre (0, -69.5) radius 3 projected
  point P0 (98.5, -74.5)
extrude "Extrusion29" add sketch "Sketch35" along normal blind 1.5
sketch "Sketch38" plane through (0, 0, 0) normal (0, 0, -1) x (-1, 0, 0)
  line L0 (-4, 81.5) -> (-4, 77) construction
  line L1 (-4, 77) -> (0.5, 77) construction
  line L2 (-4, 79.25) -> (-1.75, 79.25) construction
  line L3 (-1.75, 79.25) -> (-1.75, 77) construction
  line L4 (-1.75, 77) -> (-4, 77) construction
  line L5 (-4, 77) -> (-4, 79.25) construction
  circle A0 centre (-1.75, 79.25) radius 1.375 construction
  line L6 (-4, -0.5) -> (-4, 4) construction
  line L7 (-4, 4) -> (0.5, 4) construction
  line L8 (-1.75, 4) -> (-4, 4) construction
  line L9 (-4, 4) -> (-4, 1.75) construction
  line L10 (0.5, 18.2927) -> (0.5, 10.1927) construction
  line L11 (0.5, 1.75) -> (-1.75, 1.75) construction
  line L12 (-1.75, 1.75) -> (-1.75, -0.5) construction
  circle A1 centre (-1.75, 1.75) radius 1.375 construction
  line L13 (-124.5, -0.5) -> (-120, -0.5) construction
  line L14 (-120, -0.5) -> (-120, 4) construction
  line L15 (-120, 4) -> (-124.5, 4) construction
  line L16 (-124.5, 4) -> (-124.5, -0.5) construction
  line L17 (-122.25, 4) -> (-120, 4) construction
  line L18 (-120, 4) -> (-120, 1.75) construction
  line L19 (-120, 1.75) -> (-122.25, 1.75) construction
  line L20 (-122.25, 1.75) -> (-122.25, 4) construction
  circle A2 centre (-122.25, 1.75) radius 1.375 construction
  line L21 (-4, 4) -> (0, 4)
  line L22 (-4, 0) -> (-4, 4)
  circle A3 centre (-1.75, 1.75) radius 1.375
  circle A4 centre (-122.25, 1.75) radius 1.375
  line L23 (-120, 4) -> (-124.5, 4)
  line L24 (-124.5, 4) -> (-124.5, -0.5)
  line L25 (-124.5, -0.5) -> (-120, -0.5)
  line L26 (-120, -0.5) -> (-120, 4)
  circle A5 centre (-1.75, 79.25) radius 1.375
  line L27 (-4, 77) -> (0.5, 77)
  line L28 (0.5, 77) -> (0.5, 81.5)
  line L29 (0.5, 81.5) -> (-4, 81.5)
  line L30 (-4, 81.5) -> (-4, 77)
  line L31 (-4, 4) -> (0.5, 4)
  line L32 (0.5, 4) -> (0.5, -0.5)
  line L33 (0.5, -0.5) -> (-4, -0.5)
  line L34 (-4, -0.5) -> (-4, 4)
  line L35 (-124.5, 81.5) -> (-124.5, 77)
  line L36 (-120, 78) -> (-120, 81.5)
  line L37 (-120, 81.5) -> (-124.5, 81.5)
  line L38 (-122.25, 77) -> (-122.25, 79.25) construction
  line L39 (-122.25, 79.25) -> (-120, 79.25) construction
  circle A6 centre (-122.25, 79.25) radius 1.35
  line L40 (-121, 77) -> (-120, 78)
  line L41 (-124.5, 78.22) -> (-124.5, 72.7428) construction
  line L42 (-124.5, 81.5) -> (-124.5, 77)
  line L43 (-120, 78) -> (-120, 81.5)
  line L44 (-120, 81.5) -> (-124.5, 81.5)
  line L45 (-122.25, 77) -> (-122.25, 79.25) construction
  line L46 (-122.25, 79.25) -> (-120, 79.25) construction
  circle A7 centre (-122.25, 79.25) radius 1.35
  line L47 (-121, 77) -> (-120, 78)
  line L48 (-124.5, 78.22) -> (-124.5, 72.7428) construction
  line L49 (-124.5, 81.5) -> (-124.5, 77)
  line L50 (-120, 78) -> (-120, 81.5)
  line L51 (-120, 81.5) -> (-124.5, 81.5)
  line L52 (-122.25, 77) -> (-122.25, 79.25) construction
  line L53 (-122.25, 79.25) -> (-120, 79.25) construction
  circle A8 centre (-122.25, 79.25) radius 1.35
  line L54 (-121, 77) -> (-120, 78)
  line L55 (-124.5, 78.22) -> (-124.5, 72.7428) construction
  line L56 (-124.5, 81.5) -> (-124.5, 77)
  line L57 (-120, 78) -> (-120, 81.5)
  line L58 (-120, 81.5) -> (-124.5, 81.5)
  line L59 (-122.25, 77) -> (-122.25, 79.25) construction
  line L60 (-122.25, 79.25) -> (-120, 79.25) construction
  circle A9 centre (-122.25, 79.25) radius 1.35
  line L61 (-121, 77) -> (-120, 78)
  line L62 (-124.5, 78.22) -> (-124.5, 72.7428) construction
  line L63 (-124.5, 81.5) -> (-124.5, 77)
  line L64 (-120, 78) -> (-120, 81.5)
  line L65 (-120, 81.5) -> (-124.5, 81.5)
  line L66 (-122.25, 77) -> (-122.25, 79.25) construction
  line L67 (-122.25, 79.25) -> (-120, 79.25) construction
  circle A10 centre (-122.25, 79.25) radius 1.35
  line L68 (-121, 77) -> (-120, 78)
  line L69 (-124.5, 78.22) -> (-124.5, 72.7428) construction
  line L70 (-124.5, 77) -> (-121, 77)
  dimension "d1082" = 4.5
  dimension "d1083" = 4.5
  dimension "d1085" = 4.5
  dimension "d1086" = 4.5
  dimension "d1087" = 2.75
  dimension "d1088" = 4.5
  dimension "d1089" = 4.5
  dimension "d1090" = 2.75
  dimension "d1193" = 2.7
  dimension "d1194" = 2.7
  dimension "d1195" = 2.7
  dimension "d1196" = 2.7
  dimension "d1197" = 2.7
  constraints: 140 end point, 17 parallel, 11 centre point, 11 coincident, 9 horizontal, 7 perpendicular, 6 midpoint, 6 point on line, 3 concentric
  measures "d1082" distance of L1.end L0.end
  measures "d1083" distance of L0.end L0.start
  measures "d1085" distance of L6.end L7.end
  measures "d1086" distance of L6.start L6.end
  measures "d1087" diameter of A1
  measures "d1088" distance of L15.end L14.end
  measures "d1089" distance of L14.end L13.end
  measures "d1090" diameter of A2
  measures "d1193" diameter of A6
  measures "d1194" diameter of A7
  measures "d1195" diameter of A8
  measures "d1196" diameter of A9
  measures "d1197" diameter of A10
extrude "Extrusion32" add sketch "Sketch38" along normal blind 6.5
sketch "Sketch39" plane through (98.5, 74.5, -4.5) normal (0, 0, -1) x (-1, 0, 0)
  arc A0 (95.2784, -70.5) -> (94.5, -71.6903) centre (92.45, -69.5) ccw projected
  circle A1 centre (92.45, -69.5) radius 1.375 projected
  circle A2 centre (92.45, -69.5) radius 3
  line L0 (94.5, -71.6903) -> (94.5, -70.5) projected
  line L1 (94.5, -70.5) -> (95.2784, -70.5) projected
  point P0 (98.5, -74.5)
  constraints: 1 centre point, 1 coincident, 1 concentric
extrude "Extrusion33" cut sketch "Sketch39" along normal blind 4 contours A2 L0 L1
sketch "Sketch41" plane through (0, 0, -6.5) normal (0, 0, -1) x (-1, 0, 0)
  circle A0 centre (-1.75, 79.25) radius 1.375 construction
  circle A1 centre (-1.75, 1.75) radius 1.375 construction
  circle A2 centre (-122.25, 1.75) radius 1.375 construction
  circle A3 centre (-122.25, 1.75) radius 1.375 projected
  circle A4 centre (-1.75, 79.25) radius 1.5
  circle A5 centre (-1.75, 1.75) radius 1.5
  circle A6 centre (-122.25, 1.75) radius 1.5
  circle A7 centre (-122.25, 79.25) radius 1.35 construction
  circle A8 centre (-122.25, 79.25) radius 1.5
  point P0 (0, 0)
  dimension "d1151" = 2.75
  dimension "d1152" = 3
  dimension "d1153" = 3
  dimension "d1154" = 3
  dimension "d1198" = 3
  constraints: 4 centre point, 4 coincident
  measures "d1151" diameter of A0
  measures "d1152" diameter of A4
  measures "d1153" diameter of A5
  measures "d1154" diameter of A6
  measures "d1198" diameter of A8
extrude "Extrusion35" cut sketch "Sketch41" against normal blind 10 contours A3 | A4 | A5 | A8